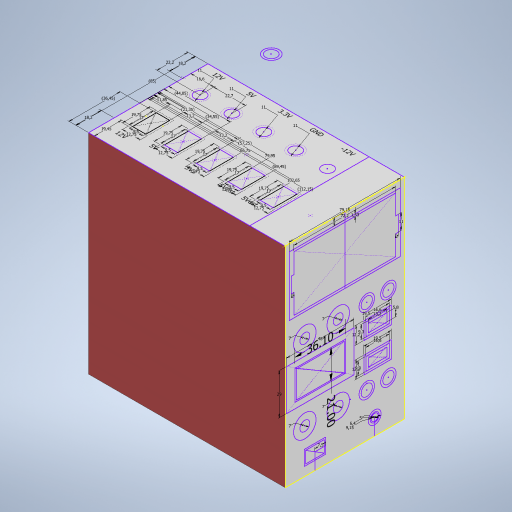
# Autodesk Inventor part: Carcasa
Saved by Autodesk Inventor 2024 (Build 280153000, 153)
## iProperties
Created: 2023-06-23
Part Number: Carcasa
Material: Genérico
Document SubType Name: Modeling
Designer: sergi
Density: 1 g/cm^3
Appearance: Valor por defecto
Author: sergi
Autodesk Inventor part; units mm, degrees
ref_plane "YZ Plane" through (0, 0, 0) normal (1, 0, 0) x (0, 1, 0)
ref_plane "XZ Plane" through (0, 0, 0) normal (0, 1, 0) x (-1, 0, 0)
ref_plane "XY Plane" through (0, 0, 0) normal (0, 0, 1) x (1, 0, 0)
sketch "Boceto1" plane through (0, 0, 0) normal (0, 1, 0) x (-1, 0, 0)
  line L0 (-70, -42.5) -> (70, -42.5)
  line L1 (70, -42.5) -> (70, 42.5)
  line L2 (70, 42.5) -> (-70, 42.5)
  line L3 (-70, 42.5) -> (-70, -42.5)
  line L4 (-70, -42.5) -> (70, 42.5) construction
  line L5 (70, -42.5) -> (-70, 42.5) construction
  point P0 (0, 0)
  dimension "d0" = 140
  dimension "d1" = 85
  constraints: 12 end point, 2 midpoint, 2 parallel, 1 horizontal, 1 perpendicular
  measures "d0" distance of L2.end L1.end
  measures "d1" distance of L1.end L0.end
extrude "Extrusión1" add sketch "Boceto1" along normal blind 149
sketch "Boceto2" plane through (70, 0, 42.5) normal (1, 0, 0) x (0, 0, -1)
  line L0 (0, 0) -> (85, 0) projected
  line L1 (85, 0) -> (85, 149) projected
  line L2 (0, 149) -> (85, 149) projected
  line L3 (0, 0) -> (0, 149) projected
  line L4 (42.5, 149) -> (42.5, 144)
  line L5 (42.5, 144) -> (42.5, 101.64)
  line L6 (42.5, 101.64) -> (82.075, 101.64)
  line L7 (82.075, 101.64) -> (2.925, 101.64)
  line L8 (2.925, 101.64) -> (2.925, 144)
  line L9 (2.925, 144) -> (82.075, 144)
  line L10 (82.075, 144) -> (82.075, 101.64)
  line L11 (78.6, 103.17) -> (6.4, 103.17)
  line L12 (6.4, 142.47) -> (78.6, 142.47)
  line L13 (78.6, 103.17) -> (6.4, 142.47) construction
  line L14 (6.4, 103.17) -> (78.6, 142.47) construction
  line L15 (78.6, 128.32) -> (80.6, 128.32)
  line L16 (80.6, 128.32) -> (80.6, 117.32)
  line L17 (80.6, 117.32) -> (78.6, 117.32)
  line L18 (6.4, 128.32) -> (4.4, 128.32)
  line L19 (4.4, 128.32) -> (4.4, 117.32)
  line L20 (4.4, 117.32) -> (6.4, 117.32)
  line L21 (6.4, 103.17) -> (6.4, 117.32)
  line L22 (6.4, 128.32) -> (6.4, 142.47)
  line L23 (78.6, 142.47) -> (78.6, 128.32)
  line L24 (78.6, 117.32) -> (78.6, 103.17)
  line L25 (85, 0) -> (85, 149) projected
  circle A0 centre (58.1, 85.17) radius 5.5
  circle A1 centre (73.5, 85.17) radius 5.5
  circle A2 centre (14, 85.17) radius 8
  circle A3 centre (14, 85.17) radius 3.5
  circle A4 centre (37.8, 85.17) radius 8
  circle A5 centre (37.8, 85.17) radius 3.5
  circle A6 centre (58.1, 85.17) radius 4
  circle A7 centre (73.5, 85.17) radius 4
  line L26 (72.4, 65.92) -> (59.2, 65.92)
  line L27 (59.2, 65.92) -> (59.2, 71.72)
  line L28 (59.2, 71.72) -> (72.4, 71.72)
  line L29 (72.4, 71.72) -> (72.4, 65.92)
  line L30 (72.4, 65.92) -> (59.2, 71.72) construction
  line L31 (59.2, 65.92) -> (72.4, 71.72) construction
  line L32 (7, 70.17) -> (43.1, 70.17)
  line L33 (43.1, 70.17) -> (43.1, 49.17)
  line L34 (43.1, 49.17) -> (7, 49.17)
  line L35 (7, 49.17) -> (7, 70.17)
  line L36 (7, 70.17) -> (43.1, 49.17)
  line L37 (42.2, 69.27) -> (7.9, 69.27)
  line L38 (7.9, 69.27) -> (7.9, 50.07)
  line L39 (7.9, 50.07) -> (42.2, 50.07)
  line L40 (42.2, 50.07) -> (42.2, 69.27)
  line L41 (42.2, 69.27) -> (7.9, 50.07) construction
  line L42 (7.9, 69.27) -> (42.2, 50.07) construction
  circle A8 centre (58.1, 31.17) radius 5.5
  circle A9 centre (73.5, 31.17) radius 5.5
  circle A10 centre (14, 31.17) radius 8
  circle A11 centre (14, 31.17) radius 3.5
  circle A12 centre (37.8, 31.17) radius 8
  circle A13 centre (37.8, 31.17) radius 3.5
  circle A14 centre (58.1, 31.17) radius 4
  circle A15 centre (73.5, 31.17) radius 4
  line L43 (28.75, 6.315) -> (13.75, 6.315)
  line L44 (13.75, 6.315) -> (13.75, 16.855)
  line L45 (13.75, 16.855) -> (28.75, 16.855)
  line L46 (28.75, 16.855) -> (28.75, 6.315)
  line L47 (28, 7.385) -> (14.5, 7.385)
  line L48 (14.5, 7.385) -> (14.5, 15.785)
  line L49 (14.5, 15.785) -> (28, 15.785)
  line L50 (28, 15.785) -> (28, 7.385)
  line L51 (72.4, 44.67) -> (72.4, 50.47)
  line L52 (59.2, 44.67) -> (72.4, 44.67)
  line L53 (59.2, 50.47) -> (72.4, 44.67) construction
  line L54 (59.2, 50.47) -> (59.2, 44.67)
  line L55 (72.4, 50.47) -> (59.2, 50.47)
  line L56 (72.4, 50.47) -> (59.2, 44.67) construction
  line L57 (14.5, 15.785) -> (28, 7.385)
  line L58 (28.75, 11.585) -> (21.25, 11.585)
  circle A16 centre (63.75, 11.585) radius 2.5
  line L59 (21.25, 11.585) -> (21.25, 0)
  line L60 (63.75, 11.585) -> (63.75, 0)
  line L61 (74.1, 64.17) -> (57.5, 64.17)
  line L62 (57.5, 64.17) -> (57.5, 73.47)
  line L63 (57.5, 73.47) -> (74.1, 73.47)
  line L64 (74.1, 73.47) -> (74.1, 64.17)
  line L65 (74.1, 64.17) -> (57.5, 73.47) construction
  line L66 (57.5, 64.17) -> (74.1, 73.47) construction
  line L67 (74.1, 42.92) -> (57.5, 42.92)
  line L68 (57.5, 42.92) -> (57.5, 52.22)
  line L69 (57.5, 52.22) -> (74.1, 52.22)
  line L70 (74.1, 52.22) -> (74.1, 42.92)
  line L71 (74.1, 42.92) -> (57.5, 52.22) construction
  line L72 (57.5, 42.92) -> (74.1, 52.22) construction
  line L73 (75.55, 62.72) -> (56.05, 62.72)
  line L74 (56.05, 62.72) -> (56.05, 74.92)
  line L75 (56.05, 74.92) -> (75.55, 74.92)
  line L76 (75.55, 74.92) -> (75.55, 62.72)
  line L77 (75.55, 62.72) -> (56.05, 74.92) construction
  line L78 (56.05, 62.72) -> (75.55, 74.92) construction
  line L79 (75.55, 41.47) -> (56.05, 41.47)
  line L80 (56.05, 41.47) -> (56.05, 53.67)
  line L81 (56.05, 53.67) -> (75.55, 53.67)
  line L82 (75.55, 53.67) -> (75.55, 41.47)
  line L83 (75.55, 41.47) -> (56.05, 53.67) construction
  line L84 (56.05, 41.47) -> (75.55, 53.67) construction
  circle A17 centre (63.75, 11.585) radius 3.2
  circle A18 centre (63.75, 11.585) radius 4.575
  line L85 (49.05, 45.17) -> (1.05, 45.17)
  line L86 (1.05, 45.17) -> (1.05, 74.17)
  line L87 (1.05, 74.17) -> (49.05, 74.17)
  line L88 (49.05, 74.17) -> (49.05, 45.17)
  line L89 (49.05, 45.17) -> (1.05, 74.17) construction
  line L90 (1.05, 45.17) -> (49.05, 74.17) construction
  point P0 (42.5, 0)
  point P1 (65.8, 68.82)
  point P2 (25.05, 59.67)
  point P3 (46.6, 31.17)
  point P4 (58.1, 35.17)
  point P5 (65.8, 47.57)
  dimension "d15" = 5
  dimension "d18" = 79.15
  dimension "d20" = 72.2
  dimension "d23" = 2
  dimension "d24" = 11
  dimension "d29" = 2
  dimension "d31" = 1.53
  dimension "d49" = 7
  dimension "d51" = 7
  dimension "d56" = 13.2
  dimension "d60" = 5.8
  dimension "d77" = 7
  dimension "d79" = 7
  dimension "d96" = 7.5
  dimension "d98" = 5
  dimension "d99" = 16.6
  dimension "d100" = 9.3
  dimension "d101" = 16.6
  dimension "d102" = 9.3
  dimension "d103" = 12.2
  dimension "d104" = 19.5
  dimension "d105" = 19.5
  dimension "d106" = 12.2
  dimension "d107" = 6.4
  dimension "d108" = 9.15
  dimension "d210" = 48
  dimension "d211" = 29
  constraints: 172 end point, 29 parallel, 19 centre point, 18 midpoint, 17 perpendicular, 14 horizontal, 10 coincident, 2 point on line
  measures "d15" distance of L4.start L4.end
  measures "d18" distance of L8.end L9.end
  measures "d20" distance of L12.start L12.end
  measures "d23" distance of L17.end L16.end
  measures "d24" distance of L15.end L16.end
  measures "d29" distance of L20.end L19.end
  measures "d31" distance between parallel lines of L12 L9
  measures "d49" diameter of A3
  measures "d51" diameter of A5
  measures "d56" distance of L27.end L28.end
  measures "d60" distance of L28.end L26.start
  measures "d77" diameter of A11
  measures "d79" diameter of A13
  measures "d96" distance of L58.start L58.end
  measures "d98" diameter of A16
  measures "d99" distance of L62.end L63.end
  measures "d100" distance of L61.end L62.end
  measures "d101" distance of L68.end L69.end
  measures "d102" distance of L67.end L68.end
  measures "d103" distance of L73.end L74.end
  measures "d104" distance of L74.end L75.end
  measures "d105" distance of L80.end L81.end
  measures "d106" distance of L79.end L80.end
  measures "d107" diameter of A17
  measures "d108" diameter of A18
  measures "d210" distance of L86.end L87.end
  measures "d211" distance of L85.end L86.end
sketch "Boceto3" plane through (0, 149, 0) normal (0, 1, 0) x (1, 0, 0)
  line L0 (-70, 42.5) -> (-70, -42.5) projected
  line L1 (-70, -42.5) -> (70, -42.5) projected
  line L2 (70, -42.5) -> (70, 42.5) projected
  line L3 (70, 42.5) -> (-70, 42.5) projected
  line L4 (70, -42.5) -> (44.8, -42.5)
  line L5 (44.8, -42.5) -> (44.8, 42.5)
  line L6 (-70, -31.6) -> (44.8, -31.6)
  line L7 (-70, -12.1) -> (44.8, -12.1)
  line L8 (-70, -42.5) -> (-70, 42.5)
  line L9 (-59.5, -12.1) -> (-47.3, -12.1)
  line L10 (-58.05, -13.55) -> (-48.75, -13.55)
  line L11 (-50.5, -15.25) -> (-56.3, -28.45) construction
  line L12 (-50.5, -28.45) -> (-56.3, -15.25) construction
  line L13 (-56.3, -28.45) -> (-56.3, -15.25)
  line L14 (-58.05, -30.15) -> (-58.05, -13.55)
  line L15 (-48.75, -30.15) -> (-58.05, -13.55) construction
  line L16 (-48.75, -13.55) -> (-58.05, -30.15) construction
  line L17 (-47.3, -31.6) -> (-59.5, -31.6)
  line L18 (-59.5, -31.6) -> (-59.5, -12.1)
  line L19 (-47.3, -12.1) -> (-59.5, -31.6) construction
  line L20 (-47.3, -31.6) -> (-59.5, -12.1) construction
  line L21 (-47.3, -12.1) -> (-47.3, -31.6)
  line L22 (-48.75, -13.55) -> (-48.75, -30.15)
  line L23 (-50.5, -28.45) -> (-56.3, -28.45)
  line L24 (-56.3, -15.25) -> (-50.5, -15.25)
  line L25 (-48.75, -30.15) -> (-58.05, -30.15)
  line L26 (-50.5, -15.25) -> (-50.5, -28.45)
  line L27 (-36.8, -12.1) -> (-24.6, -12.1)
  line L28 (-35.35, -13.55) -> (-26.05, -13.55)
  line L29 (-27.8, -15.25) -> (-33.6, -28.45) construction
  line L30 (-27.8, -28.45) -> (-33.6, -15.25) construction
  line L31 (-33.6, -28.45) -> (-33.6, -15.25)
  line L32 (-35.35, -30.15) -> (-35.35, -13.55)
  line L33 (-26.05, -30.15) -> (-35.35, -13.55) construction
  line L34 (-26.05, -13.55) -> (-35.35, -30.15) construction
  line L35 (-24.6, -31.6) -> (-36.8, -31.6)
  line L36 (-36.8, -31.6) -> (-36.8, -12.1)
  line L37 (-24.6, -12.1) -> (-36.8, -31.6) construction
  line L38 (-24.6, -31.6) -> (-36.8, -12.1) construction
  line L39 (-24.6, -12.1) -> (-24.6, -31.6)
  line L40 (-26.05, -13.55) -> (-26.05, -30.15)
  line L41 (-27.8, -28.45) -> (-33.6, -28.45)
  line L42 (-33.6, -15.25) -> (-27.8, -15.25)
  line L43 (-26.05, -30.15) -> (-35.35, -30.15)
  line L44 (-27.8, -15.25) -> (-27.8, -28.45)
  line L45 (-13.8, -12.1) -> (-1.6, -12.1)
  line L46 (-12.35, -13.55) -> (-3.05, -13.55)
  line L47 (-4.8, -15.25) -> (-10.6, -28.45) construction
  line L48 (-4.8, -28.45) -> (-10.6, -15.25) construction
  line L49 (-10.6, -28.45) -> (-10.6, -15.25)
  line L50 (-12.35, -30.15) -> (-12.35, -13.55)
  line L51 (-3.05, -30.15) -> (-12.35, -13.55) construction
  line L52 (-3.05, -13.55) -> (-12.35, -30.15) construction
  line L53 (-1.6, -31.6) -> (-13.8, -31.6)
  line L54 (-13.8, -31.6) -> (-13.8, -12.1)
  line L55 (-1.6, -12.1) -> (-13.8, -31.6) construction
  line L56 (-1.6, -31.6) -> (-13.8, -12.1) construction
  line L57 (-1.6, -12.1) -> (-1.6, -31.6)
  line L58 (-3.05, -13.55) -> (-3.05, -30.15)
  line L59 (-4.8, -28.45) -> (-10.6, -28.45)
  line L60 (-10.6, -15.25) -> (-4.8, -15.25)
  line L61 (-3.05, -30.15) -> (-12.35, -30.15)
  line L62 (-4.8, -15.25) -> (-4.8, -28.45)
  circle A0 centre (-53.4, 4.3) radius 4
  circle A1 centre (-53.4, 4.3) radius 5.5
  circle A2 centre (-53.4, 19.7) radius 4
  circle A3 centre (-53.4, 19.7) radius 5.5
  circle A4 centre (-30.7, 4.3) radius 4
  circle A5 centre (-30.7, 4.3) radius 5.5
  circle A6 centre (-30.7, 19.7) radius 4
  circle A7 centre (-30.7, 19.7) radius 5.5
  circle A8 centre (-8, 4.3) radius 4
  circle A9 centre (-8, 4.3) radius 5.5
  circle A10 centre (-8, 19.7) radius 4
  circle A11 centre (-8, 19.7) radius 5.5
  line L63 (-1.6, -31.6) -> (8.9, -31.6)
  line L64 (8.9, -31.6) -> (21.1, -31.6)
  line L65 (21.1, -31.6) -> (31.6, -31.6)
  line L66 (11.6788, -28.45) -> (17.4788, -28.45)
  line L67 (17.4788, -28.45) -> (17.4788, -15.25)
  line L68 (19.2288, -13.55) -> (19.2288, -30.15)
  line L69 (20.6788, -12.1) -> (20.6788, -31.6)
  line L70 (19.2288, -30.15) -> (9.9288, -30.15)
  line L71 (20.6788, -31.6) -> (8.4788, -31.6)
  line L72 (11.6788, -15.25) -> (17.4788, -28.45) construction
  line L73 (11.6788, -28.45) -> (17.4788, -15.25) construction
  line L74 (11.6788, -15.25) -> (11.6788, -28.45)
  line L75 (9.9288, -30.15) -> (9.9288, -13.55)
  line L76 (19.2288, -30.15) -> (9.9288, -13.55) construction
  line L77 (19.2288, -13.55) -> (9.9288, -30.15) construction
  line L78 (8.4788, -31.6) -> (8.4788, -12.1)
  line L79 (20.6788, -12.1) -> (8.4788, -31.6) construction
  line L80 (20.6788, -31.6) -> (8.4788, -12.1) construction
  line L81 (17.4788, -15.25) -> (11.6788, -15.25)
  line L82 (9.9288, -13.55) -> (19.2288, -13.55)
  line L83 (8.4788, -12.1) -> (20.6788, -12.1)
  line L84 (34.8, -28.45) -> (40.6, -28.45)
  line L85 (40.6, -28.45) -> (40.6, -15.25)
  line L86 (42.35, -13.55) -> (42.35, -30.15)
  line L87 (43.8, -12.1) -> (43.8, -31.6)
  line L88 (42.35, -30.15) -> (33.05, -30.15)
  line L89 (43.8, -31.6) -> (31.6, -31.6)
  line L90 (34.8, -15.25) -> (40.6, -28.45) construction
  line L91 (34.8, -28.45) -> (40.6, -15.25) construction
  line L92 (34.8, -15.25) -> (34.8, -28.45)
  line L93 (33.05, -30.15) -> (33.05, -13.55)
  line L94 (42.35, -30.15) -> (33.05, -13.55) construction
  line L95 (42.35, -13.55) -> (33.05, -30.15) construction
  line L96 (31.6, -31.6) -> (31.6, -12.1)
  line L97 (43.8, -12.1) -> (31.6, -31.6) construction
  line L98 (43.8, -31.6) -> (31.6, -12.1) construction
  line L99 (40.6, -15.25) -> (34.8, -15.25)
  line L100 (33.05, -13.55) -> (42.35, -13.55)
  line L101 (31.6, -12.1) -> (43.8, -12.1)
  line L102 (42.35, 30.15) -> (42.35, 13.55)
  line L103 (43.8, 31.6) -> (43.8, 12.1)
  line L104 (42.35, 13.55) -> (33.05, 13.55)
  line L105 (43.8, 12.1) -> (31.6, 12.1)
  line L106 (33.05, 13.55) -> (33.05, 30.15)
  line L107 (42.35, 13.55) -> (33.05, 30.15) construction
  line L108 (42.35, 30.15) -> (33.05, 13.55) construction
  line L109 (31.6, 12.1) -> (31.6, 31.6)
  line L110 (43.8, 31.6) -> (31.6, 12.1) construction
  line L111 (43.8, 12.1) -> (31.6, 31.6) construction
  line L112 (33.05, 30.15) -> (42.35, 30.15)
  line L113 (31.6, 31.6) -> (43.8, 31.6)
  line L114 (19.2288, 30.15) -> (19.2288, 13.55)
  line L115 (20.6788, 31.6) -> (20.6788, 12.1)
  line L116 (19.2288, 13.55) -> (9.9288, 13.55)
  line L117 (20.6788, 12.1) -> (8.4788, 12.1)
  line L118 (9.9288, 13.55) -> (9.9288, 30.15)
  line L119 (19.2288, 13.55) -> (9.9288, 30.15) construction
  line L120 (19.2288, 30.15) -> (9.9288, 13.55) construction
  line L121 (8.4788, 12.1) -> (8.4788, 31.6)
  line L122 (20.6788, 31.6) -> (8.4788, 12.1) construction
  line L123 (20.6788, 12.1) -> (8.4788, 31.6) construction
  line L124 (9.9288, 30.15) -> (19.2288, 30.15)
  line L125 (8.4788, 31.6) -> (20.6788, 31.6)
  line L126 (-70, 25.2) -> (-70, 42.5)
  point P0 (0, 0)
  point P1 (-53.4, -21.85)
  point P2 (-30.7, -21.85)
  point P3 (-7.7, -21.85)
  point P4 (14.5788, -21.85)
  point P5 (37.7, -21.85)
  point P6 (37.7, 21.85)
  point P7 (14.5788, 21.85)
  point P8 (-53.4, -12.1)
  dimension "d119" = 25.2
  dimension "d124" = 19.5
  dimension "d141" = 13.2
  dimension "d142" = 5.8
  dimension "d144" = 9.3
  dimension "d145" = 12.2
  dimension "d146" = 19.5
  dimension "d147" = 13.2
  dimension "d148" = 5.8
  dimension "d149" = 16.6
  dimension "d150" = 9.3
  dimension "d151" = 12.2
  dimension "d152" = 19.5
  dimension "d162" = 10.8
  dimension "d176" = 10.5
  dimension "d177" = 12.2
  dimension "d179" = 16.6
  dimension "d180" = 9.3
  dimension "d181" = 19.5
  dimension "d182" = 12.2
  dimension "d183" = 16.6
  dimension "d184" = 9.3
  dimension "d185" = 19.5
  dimension "d186" = 12.2
  dimension "d187" = 16.6
  dimension "d188" = 9.3
  dimension "d189" = 19.5
  dimension "d190" = 12.2
  dimension "d191" = 16.6
  dimension "d192" = 9.3
  dimension "d193" = 19.5
  dimension "d194" = 12.2
  dimension "d201" = 10.9
  dimension "d202" = 10.9
  dimension "d203" = 10.9
  constraints: 246 end point, 35 midpoint, 35 parallel, 18 perpendicular, 12 centre point, 6 coincident, 5 point on line, 1 collinear, 1 vertical
  measures "d119" distance of L1.end L4.end
  measures "d124" distance between parallel lines of L6 L7
  measures "d141" distance of L31.start L31.end
  measures "d142" distance of L31.end L44.start
  measures "d144" distance of L43.start L43.end
  measures "d145" distance of L35.start L35.end
  measures "d146" distance of L35.end L27.start
  measures "d147" distance of L49.start L49.end
  measures "d148" distance of L49.end L62.start
  measures "d149" distance of L61.end L46.start
  measures "d150" distance of L61.start L61.end
  measures "d151" distance of L53.start L53.end
  measures "d152" distance of L53.end L45.start
  measures "d162" distance between parallel lines of L54 L39
  measures "d176" distance of L53.start L63.end
  measures "d177" distance of L63.end L64.end
  measures "d179" distance of L77.end L82.start
  measures "d180" distance of L68.end L77.end
  measures "d181" distance of L79.end L83.start
  measures "d182" distance of L80.start L79.end
  measures "d183" distance of L95.end L100.start
  measures "d184" distance of L86.end L95.end
  measures "d185" distance of L97.end L101.start
  measures "d186" distance of L98.start L97.end
  measures "d187" distance of L108.end L112.start
  measures "d188" distance of L102.end L108.end
  measures "d189" distance of L110.end L113.start
  measures "d190" distance of L103.end L110.end
  measures "d191" distance of L120.end L124.start
  measures "d192" distance of L114.end L120.end
  measures "d193" distance of L122.end L125.start
  measures "d194" distance of L115.end L122.end
  measures "d201" distance between parallel lines of L1 L64
  measures "d202" distance between parallel lines of L3 L125
  measures "d203" distance between parallel lines of L3 L113
sketch "Boceto5" plane through (0, 149, 0) normal (0, 1, 0) x (1, 0, 0)
  line L0 (-70, 42.5) -> (-70, -42.5)
  line L1 (-70, 42.5) -> (-70, -42.5)
  line L2 (-70, -42.5) -> (70, -42.5)
  line L3 (-70, -42.5) -> (70, -42.5)
  line L4 (70, 42.5) -> (-70, 42.5)
  line L5 (70, 42.5) -> (-70, 42.5)
  line L6 (-70, 42.5) -> (-70, -42.5)
  line L7 (70, 42.5) -> (-70, 42.5)
  line L8 (-70, -42.5) -> (70, -42.5)
  line L9 (-70, 42.5) -> (-70, -42.5)
  line L10 (-70, -42.5) -> (70, -42.5)
  line L11 (70, 42.5) -> (-70, 42.5)
  line L12 (-70, 42.5) -> (-70, -42.5)
  line L13 (-70, 42.5) -> (-70, -42.5)
  line L14 (-70, -42.5) -> (70, -42.5)
  line L15 (-70, -42.5) -> (70, -42.5)
  line L16 (70, 42.5) -> (-70, 42.5)
  line L17 (70, 42.5) -> (-70, 42.5)
  line L18 (-70, -42.5) -> (70, -42.5)
  line L19 (70, 42.5) -> (-70, 42.5)
  line L20 (44.8, -42.5) -> (44.8, 42.5)
  line L21 (-70, 42.5) -> (-70, -42.5)
  line L22 (-70, -42.5) -> (-70, 42.5)
  line L23 (-70, 25.2) -> (-70, 42.5)
  line L24 (70, -42.5) -> (44.8, -42.5)
  line L25 (44.8, -42.5) -> (44.8, 42.5)
  circle A0 centre (-53.4, 71) radius 4
  circle A1 centre (-53.4, 71) radius 5.5
  line L26 (-70, -42.5) -> (-70, -24.3)
  line L27 (-70, 42.5) -> (-70, 24.3)
  circle A2 centre (-53.4, 20.3) radius 4
  circle A3 centre (-53.4, 20.3) radius 5.5 construction
  circle A4 centre (-30.7, 20.3) radius 4
  circle A5 centre (-30.7, 20.3) radius 5.5 construction
  circle A6 centre (-8, 20.3) radius 4
  circle A7 centre (-8, 20.3) radius 5.5 construction
  circle A8 centre (14.7, 20.3) radius 4
  circle A9 centre (14.7, 20.3) radius 5.5 construction
  circle A10 centre (37.4, 20.3) radius 4
  line L28 (-61.8165, 40.0405) -> (-42.6105, 40.0405) construction
  line L29 (-42.6105, 40.0405) -> (-42.6105, 31.8343) construction
  line L30 (-42.6105, 31.8343) -> (-61.8165, 31.8343) construction
  line L31 (-61.8165, 31.8343) -> (-61.8165, 40.0405) construction
  line L32 (-37.7217, 40.2151) -> (-19.0395, 40.2151) construction
  line L33 (-19.0395, 40.2151) -> (-19.0395, 32.7073) construction
  line L34 (-19.0395, 32.7073) -> (-37.7217, 32.7073) construction
  line L35 (-37.7217, 32.7073) -> (-37.7217, 40.2151) construction
  line L36 (-15.7221, 40.7389) -> (2.7855, 40.7389) construction
  line L37 (2.7855, 40.7389) -> (2.7855, 32.5327) construction
  line L38 (2.7855, 32.5327) -> (-15.7221, 32.5327) construction
  line L39 (-15.7221, 32.5327) -> (-15.7221, 40.7389) construction
  line L40 (6.9759, 40.5643) -> (26.1819, 40.5643) construction
  line L41 (26.1819, 40.5643) -> (26.1819, 32.1835) construction
  line L42 (26.1819, 32.1835) -> (6.9759, 32.1835) construction
  line L43 (6.9759, 32.1835) -> (6.9759, 40.5643) construction
  line L44 (29.8485, 39.6913) -> (42.7689, 39.6913) construction
  line L45 (42.7689, 39.6913) -> (42.7689, 32.0089) construction
  line L46 (42.7689, 32.0089) -> (29.8485, 32.0089) construction
  line L47 (29.8485, 32.0089) -> (29.8485, 39.6913) construction
  line L48 (-60.4197, -30.4979) -> (-46.4517, -30.4979) construction
  line L49 (-46.4517, -30.4979) -> (-46.4517, -37.6565) construction
  line L50 (-46.4517, -37.6565) -> (-60.4197, -37.6565) construction
  line L51 (-60.4197, -37.6565) -> (-60.4197, -30.4979) construction
  line L52 (-40.1661, -26.4821) -> (-17.6427, -26.4821) construction
  line L53 (-17.6427, -26.4821) -> (-17.6427, -37.6565) construction
  line L54 (-17.6427, -37.6565) -> (-40.1661, -37.6565) construction
  line L55 (-40.1661, -37.6565) -> (-40.1661, -26.4821) construction
  line L56 (-13.9761, -27.3551) -> (10.8171, -27.3551) construction
  line L57 (10.8171, -27.3551) -> (10.8171, -36.0851) construction
  line L58 (10.8171, -36.0851) -> (-13.9761, -36.0851) construction
  line L59 (-13.9761, -36.0851) -> (-13.9761, -27.3551) construction
  line L60 (8.8965, -26.3075) -> (26.8803, -26.3075) construction
  line L61 (26.8803, -26.3075) -> (26.8803, -35.2121) construction
  line L62 (26.8803, -35.2121) -> (8.8965, -35.2121) construction
  line L63 (8.8965, -35.2121) -> (8.8965, -26.3075) construction
  line L64 (24.7851, -25.9583) -> (44.6895, -25.9583) construction
  line L65 (44.6895, -25.9583) -> (44.6895, -35.2121) construction
  line L66 (44.6895, -35.2121) -> (24.7851, -35.2121) construction
  line L67 (24.7851, -35.2121) -> (24.7851, -25.9583) construction
  line L68 (-47.025, -4.675) -> (-59.775, -4.675) construction
  line L69 (-59.775, -4.675) -> (-59.775, -24.425) construction
  line L70 (-59.775, -24.425) -> (-47.025, -24.425) construction
  line L71 (-47.025, -24.425) -> (-47.025, -4.675) construction
  line L72 (-47.025, -24.425) -> (-59.775, -4.675) construction
  line L73 (-48.65, -6.05) -> (-58.15, -6.05)
  line L74 (-58.15, -6.05) -> (-58.15, -23.05)
  line L75 (-58.15, -23.05) -> (-48.65, -23.05)
  line L76 (-48.65, -23.05) -> (-48.65, -6.05)
  line L77 (-48.65, -6.05) -> (-58.15, -23.05) construction
  line L78 (-58.15, -6.05) -> (-48.65, -23.05) construction
  line L79 (-24.325, -4.675) -> (-37.075, -4.675) construction
  line L80 (-37.075, -4.675) -> (-37.075, -24.425) construction
  line L81 (-37.075, -24.425) -> (-24.325, -24.425) construction
  line L82 (-24.325, -24.425) -> (-24.325, -4.675) construction
  line L83 (-24.325, -24.425) -> (-37.075, -4.675) construction
  line L84 (-25.95, -6.05) -> (-35.45, -6.05)
  line L85 (-35.45, -6.05) -> (-35.45, -23.05)
  line L86 (-35.45, -23.05) -> (-25.95, -23.05)
  line L87 (-25.95, -23.05) -> (-25.95, -6.05)
  line L88 (-25.95, -6.05) -> (-35.45, -23.05) construction
  line L89 (-35.45, -6.05) -> (-25.95, -23.05) construction
  line L90 (-1.625, -4.675) -> (-14.375, -4.675) construction
  line L91 (-14.375, -4.675) -> (-14.375, -24.425) construction
  line L92 (-14.375, -24.425) -> (-1.625, -24.425) construction
  line L93 (-1.625, -24.425) -> (-1.625, -4.675) construction
  line L94 (-1.625, -24.425) -> (-14.375, -4.675) construction
  line L95 (-3.25, -6.05) -> (-12.75, -6.05)
  line L96 (-12.75, -6.05) -> (-12.75, -23.05)
  line L97 (-12.75, -23.05) -> (-3.25, -23.05)
  line L98 (-3.25, -23.05) -> (-3.25, -6.05)
  line L99 (-3.25, -6.05) -> (-12.75, -23.05) construction
  line L100 (-12.75, -6.05) -> (-3.25, -23.05) construction
  line L101 (21.075, -4.675) -> (8.325, -4.675) construction
  line L102 (8.325, -4.675) -> (8.325, -24.425) construction
  line L103 (8.325, -24.425) -> (21.075, -24.425) construction
  line L104 (21.075, -24.425) -> (21.075, -4.675) construction
  line L105 (21.075, -24.425) -> (8.325, -4.675) construction
  line L106 (19.45, -6.05) -> (9.95, -6.05)
  line L107 (9.95, -6.05) -> (9.95, -23.05)
  line L108 (9.95, -23.05) -> (19.45, -23.05)
  line L109 (19.45, -23.05) -> (19.45, -6.05)
  line L110 (19.45, -6.05) -> (9.95, -23.05) construction
  line L111 (9.95, -6.05) -> (19.45, -23.05) construction
  line L112 (43.775, -4.675) -> (31.025, -4.675) construction
  line L113 (31.025, -4.675) -> (31.025, -24.425) construction
  line L114 (31.025, -24.425) -> (43.775, -24.425) construction
  line L115 (43.775, -24.425) -> (43.775, -4.675) construction
  line L116 (43.775, -24.425) -> (31.025, -4.675) construction
  line L117 (42.15, -6.05) -> (32.65, -6.05)
  line L118 (32.65, -6.05) -> (32.65, -23.05)
  line L119 (32.65, -23.05) -> (42.15, -23.05)
  line L120 (42.15, -23.05) -> (42.15, -6.05)
  line L121 (42.15, -6.05) -> (32.65, -23.05) construction
  line L122 (32.65, -6.05) -> (42.15, -23.05) construction
  point P0 (70, 39.575)
  point P1 (70, 36.1)
  point P2 (70, 36.1)
  point P3 (70, 38.1)
  point P4 (70, 36.1)
  point P5 (70, 38.1)
  point P6 (70, 36.1)
  point P7 (70, 39.575)
  point P8 (70, -32)
  point P9 (70, -25)
  point P10 (70, -36.5)
  point P11 (70, -20.5)
  point P12 (70, -12.7)
  point P13 (70, 3.3)
  point P14 (70, 0.6)
  point P15 (70, -0.3)
  point P16 (70, -8.2)
  point P17 (70, -1.2)
  point P18 (70, 6.55)
  point P19 (70, -0.3)
  point P20 (70, 0.6)
  point P21 (70, 6.55)
  point P22 (70, -34.6)
  point P23 (70, -35.5)
  point P24 (70, -34.6)
  point P25 (70, -35.5)
  point P26 (70, -41.45)
  point P27 (70, -41.45)
  point P28 (70, 10.1)
  point P29 (70, 21.1)
  point P30 (70, 25.5)
  point P31 (70, 36.5)
  point P32 (70, 11.6)
  point P33 (70, 19.6)
  point P34 (70, 27)
  point P35 (70, 35)
  point P36 (70, 15)
  point P37 (70, 31.6)
  point P38 (70, 15)
  point P39 (70, 31.6)
  point P40 (70, 13.55)
  point P41 (70, 13.55)
  point P42 (70, 33.05)
  point P43 (70, 33.05)
  point P44 (70, 15)
  point P45 (70, 31.6)
  point P46 (70, 29.9)
  point P47 (70, 16.7)
  point P48 (70, 16.7)
  point P49 (70, 29.9)
  point P50 (70, 29.9)
  point P51 (70, 16.7)
  point P52 (70, 29.9)
  point P53 (70, 16.7)
  point P54 (70, 13.55)
  point P55 (70, 33.05)
  point P56 (70, 15)
  point P57 (70, 31.6)
  point P58 (70, 33.05)
  point P59 (70, 13.55)
  point P60 (70, 0)
  point P61 (70, -36.1)
  point P62 (70, -39.575)
  point P63 (70, -36.1)
  point P64 (70, -38.1)
  point P65 (70, -38.1)
  point P66 (70, -36.1)
  point P67 (70, -36.1)
  point P68 (70, -39.575)
  point P69 (70, -13.75)
  point P70 (70, -13.75)
  point P71 (70, -13.75)
  point P72 (70, -14.5)
  point P73 (70, -14.5)
  point P74 (70, -21.25)
  point P75 (70, -28)
  point P76 (70, -28.75)
  point P77 (70, -28)
  point P78 (70, -28.75)
  point P79 (0, 0)
  point P80 (-70, -12.1)
  point P81 (-59.5, -12.1)
  point P82 (-47.3, -12.1)
  point P83 (-30.7, -14.55)
  point P84 (-53.4, -14.55)
  point P85 (-8, -14.55)
  point P86 (-30.7, -14.55)
  point P87 (14.7, -14.55)
  point P88 (-8, -14.55)
  point P89 (37.4, -14.55)
  point P90 (14.7, -14.55)
  point P91 (60.1, -14.55)
  point P92 (37.4, -14.55)
  dimension "d215" = 85
  dimension "d218" = 18.2
  dimension "d219" = 18.2
  dimension "d225" = 11
  dimension "d226" = 11
  dimension "d227" = 11
  dimension "d228" = 11
  dimension "d237" = 12.75
  dimension "d238" = 19.75
  dimension "d240" = 9.5
  dimension "d241" = 17
  dimension "d246" = 12.75
  dimension "d247" = 19.75
  dimension "d248" = 9.5
  dimension "d249" = 17
  dimension "d250" = 12.75
  dimension "d251" = 19.75
  dimension "d252" = 9.5
  dimension "d253" = 17
  dimension "d254" = 12.75
  dimension "d255" = 19.75
  dimension "d256" = 9.5
  dimension "d257" = 17
  dimension "d258" = 12.75
  dimension "d259" = 19.75
  dimension "d260" = 9.5
  dimension "d261" = 17
  dimension "d262" = 11.85
  dimension "d263" = 13.2
  dimension "d264" = 13.2
  dimension "d265" = 19.45
  dimension "d266" = 36.45
  dimension "d267" = 21.35
  dimension "d268" = 34.55
  dimension "d269" = 44.05
  dimension "d270" = 57.25
  dimension "d271" = 66.75
  dimension "d272" = 79.95
  dimension "d273" = 89.45
  dimension "d274" = 102.65
  dimension "d275" = 112.15
  dimension "d276" = 16.6
  dimension "d277" = 22.2
  dimension "d278" = 22.7
  constraints: 154 end point, 20 parallel, 15 midpoint, 11 centre point, 10 horizontal, 10 perpendicular, 40 other
  measures "d215" distance of L0.start L0.end
  measures "d218" distance of L26.start L26.end
  measures "d219" distance of L27.start L27.end
  measures "d225" diameter of A3
  measures "d226" diameter of A5
  measures "d227" diameter of A7
  measures "d228" diameter of A9
  measures "d237" distance of L70.end L69.end
  measures "d238" distance of L69.end L68.end
  measures "d240" distance of L75.end L74.end
  measures "d241" distance of L74.end L73.end
  measures "d246" distance of L82.start L80.end
  measures "d247" distance of L80.end L79.end
  measures "d248" distance of L87.start L86.start
  measures "d249" distance of L86.start L84.end
  measures "d250" distance of L93.start L91.end
  measures "d251" distance of L91.end L90.end
  measures "d252" distance of L98.start L97.start
  measures "d253" distance of L97.start L95.end
  measures "d254" distance of L104.start L102.end
  measures "d255" distance of L102.end L101.end
  measures "d256" distance of L109.start L108.start
  measures "d257" distance of L108.start L106.end
  measures "d258" distance of L115.start L113.end
  measures "d259" distance of L113.end L112.end
  measures "d260" distance of L120.start L119.start
  measures "d261" distance of L119.start L117.end
  measures "d262" distance between parallel lines of L13 L74
  measures "d263" distance between parallel lines of L85 L76
  measures "d264" distance between parallel lines of L96 L87
  measures "d265" distance between parallel lines of L8 L75
  measures "d266" distance between parallel lines of L73 L8
  measures "d267" distance between parallel lines of L76 L13
  measures "d268" distance between parallel lines of L85 L13
  measures "d269" distance between parallel lines of L13 L87
  measures "d270" distance between parallel lines of L96 L13
  measures "d272" distance between parallel lines of L107 L0
  measures "d275" distance between parallel lines of L120 L6
  measures "d277" distance from line of L4 A2.centre
  measures "d278" distance of A4.centre A2.centre
